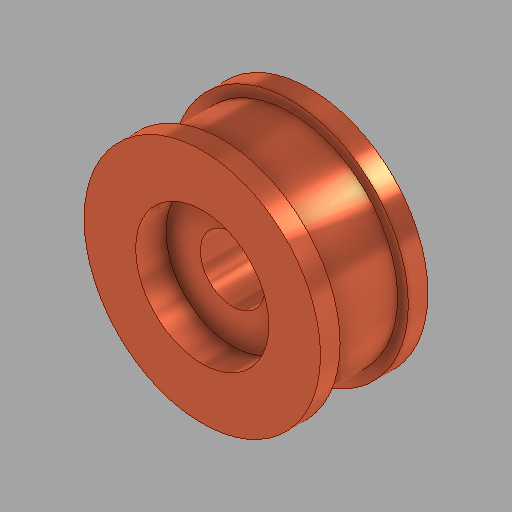
# Autodesk Inventor part: Rodillo Guia de Cadena
Saved by Autodesk Inventor 2024.3 (Build 283343010, 343A)
## iProperties
Created: 2025-05-04
Part Number: Rodillo Guia de Cadena
Material: Steel, Galvanized
Document SubType Name: Modeling
Designer: Gary
Density: 7.85 g/cm^3
Appearance: Metal 1400F Hot
Author: Gary
Autodesk Inventor part; units mm, degrees
ref_plane "YZ Plane" through (0, 0, 0) normal (1, 0, 0) x (0, 1, 0)
ref_plane "XZ Plane" through (0, 0, 0) normal (0, 1, 0) x (-1, 0, 0)
sketch "Sketch1" plane through (0, 0, 0) normal (0, 0, 1) x (1, 0, 0)
  circle A0 centre (0, 0) radius 31
  circle A1 centre (0, 0) radius 55
  dimension "d0" = 62
  dimension "d1" = 110
  constraints: 2 centre point, 2 coincident
  measures "d0" diameter of A0
  measures "d1" diameter of A1
extrude "Extrusion1" add sketch "Sketch1" along normal blind 9.12
sketch "Sketch2" plane through (0, 0, 9.12) normal (0, 0, 1) x (1, 0, 0)
  circle A0 centre (0, 0) radius 50
  circle A1 centre (0, 0) radius 15
  dimension "d4" = 100
  dimension "d5" = 30
  constraints: 2 centre point, 2 coincident
  measures "d4" diameter of A0
  measures "d5" diameter of A1
extrude "Extrusion2" add sketch "Sketch2" along normal blind 31.76
ref_plane "Work Plane1" through (0, 0, 25) normal (0, 0, 1) x (1, 0, 0)
sketch "Sketch3" plane through (0, 0, 9.12) normal (0, 0, -1) x (-1, 0, 0)
  circle A0 centre (0, 0) radius 31 projected
  circle A1 centre (0, 0) radius 31
  dimension "d8" = 62
  constraints: 1 centre point, 1 coincident
  measures "d8" diameter of A1
extrude "Extrusion3" cut sketch "Sketch3" against normal blind 5
mirror "Mirror1" about plane through (0, 0, 25) normal (0, 0, 1) of "Extrusion1", "Extrusion3", "Extrusion2"
sketch "Sketch4" plane through (0, 0, 9.12) normal (0, 0, -1) x (-1, 0, 0)
  circle A0 centre (0, 0) radius 31
  dimension "d11" = 62
  constraints: 1 centre point, 1 coincident
  measures "d11" diameter of A0
extrude "Extrusion4" cut sketch "Sketch4" against normal blind 5
body "Solid1"
